Autodesk Inventor part; units mm, degrees
(part 3 of 3)
  line L522 (9.5, 12.75) -> (20, 12.75)
  line L523 (20, 12.75) -> (20, -5.25)
  line L524 (20, -5.25) -> (9.5, -5.25)
  line L525 (9.5, -5.25) -> (9.5, 12.75)
  line L526 (9.5, 17.25) -> (20, 17.25)
  line L527 (20, 17.25) -> (20, 35.25)
  line L528 (20, 35.25) -> (9.5, 35.25)
  line L529 (9.5, 35.25) -> (9.5, 17.25)
  line L530 (9.5, 57.75) -> (20, 57.75)
  line L531 (20, 57.75) -> (20, 39.75)
  line L532 (20, 39.75) -> (9.5, 39.75)
  line L533 (9.5, 39.75) -> (9.5, 57.75)
  line L534 (9.5, 62.25) -> (20, 62.25)
  line L535 (20, 62.25) -> (20, 80.25)
  line L536 (20, 80.25) -> (9.5, 80.25)
  line L537 (9.5, 80.25) -> (9.5, 62.25)
  line L538 (9.5, 117.75) -> (20, 117.75)
  line L539 (20, 117.75) -> (20, 99.75)
  line L540 (20, 99.75) -> (9.5, 99.75)
  line L541 (9.5, 99.75) -> (9.5, 117.75)
  line L542 (9.5, 84.75) -> (20, 84.75)
  line L543 (20, 84.75) -> (20, 95.25)
  line L544 (20, 95.25) -> (9.5, 95.25)
  line L545 (9.5, 95.25) -> (9.5, 84.75)
  point P0 (0, 0)
  point P1 (9.5, -64.25)
  point P2 (20, -53.75)
  point P3 (20, -49.25)
  point P4 (20, -8.75)
  point P5 (20, -4.25)
  point P6 (20, 36.25)
  point P7 (9.5, 40.75)
  point P8 (20, 51.25)
  point P9 (20, 55.75)
  point P10 (20, 96.25)
  point P11 (20, 100.75)
  point P12 (35, 27.75)
  point P13 (35, 17.25)
  point P14 (39.5, 17.25)
  point P15 (39.5, 27.75)
  point P16 (35, 42.75)
  point P17 (35, 57.75)
  point P18 (35, 72.75)
  point P19 (35, -47.25)
  point P20 (35, -77.25)
  point P21 (35, -32.25)
  point P22 (39.5, -32.25)
  point P23 (35, -17.25)
  point P24 (39.5, -17.25)
  point P25 (39.5, -12.75)
  point P26 (39.5, -2.25)
  point P27 (35, 12.75)
  point P28 (35, 2.25)
  point P29 (39.5, 2.25)
  point P30 (39.5, 12.75)
  point P31 (9.5, 99.75)
  point P32 (20, 99.75)
  point P33 (20, 102.75)
  point P34 (20, 107.25)
  point P35 (9.5, 107.25)
  point P36 (9.5, 102.75)
  point P37 (9.5, 95.25)
  point P38 (9.5, 92.25)
  point P39 (9.5, 87.75)
  point P40 (20, 84.75)
  point P41 (20, 87.75)
  point P42 (20, 92.25)
  point P43 (9.5, 80.25)
  point P44 (9.5, 77.25)
  point P45 (9.5, 72.75)
  point P46 (20, 72.75)
  point P47 (20, 77.25)
  point P48 (9.5, 39.75)
  point P49 (20, 42.75)
  point P50 (20, 47.25)
  point P51 (9.5, 47.25)
  point P52 (9.5, 42.75)
  point P53 (20, 35.25)
  point P54 (9.5, 35.25)
  point P55 (9.5, 32.25)
  point P56 (9.5, 27.75)
  point P57 (20, 27.75)
  point P58 (20, 32.25)
  point P59 (9.5, -5.25)
  point P60 (20, -5.25)
  point P61 (20, -2.25)
  point P62 (20, 2.25)
  point P63 (9.5, 2.25)
  point P64 (9.5, -2.25)
  point P65 (9.5, -9.75)
  point P66 (9.5, -12.75)
  point P67 (9.5, -17.25)
  point P68 (20, -20.25)
  point P69 (20, -17.25)
  point P70 (20, -12.75)
  point P71 (9.5, -24.75)
  point P72 (9.5, -27.75)
  point P73 (9.5, -32.25)
  point P74 (20, -32.25)
  point P75 (20, -27.75)
  point P76 (9.5, -65.25)
  point P77 (20, -62.25)
  point P78 (20, -57.75)
  point P79 (9.5, -57.75)
  point P80 (9.5, -62.25)
  point P81 (9.5, -69.75)
  point P82 (9.5, -72.75)
  point P83 (9.5, -77.25)
  point P84 (20, -77.25)
  point P85 (20, -72.75)
  dimension "d223" = 0.25
  dimension "d224" = 10.5
  dimension "d225" = 10.5
  dimension "d226" = 0.25
  dimension "d229" = 15
  dimension "d232" = 15
  dimension "d283" = 10.5
  dimension "d284" = 18
  dimension "d285" = 18
  dimension "d286" = 18
  dimension "d287" = 10.5
  dimension "d288" = 4.5
  dimension "d289" = 18
  dimension "d290" = 18
  dimension "d291" = 18
  dimension "d292" = 18
  dimension "d293" = 18
  dimension "d294" = 10.5
  dimension "d295" = 4.5
  constraints: 1088 end point, 50 parallel, 26 horizontal, 25 perpendicular, 21 point on line, 2 collinear, 1 vertical, 886 other
  measures "d223" distance between parallel lines of L4 L0
  measures "d224" distance of L0.start L0.end
  measures "d225" distance of L0.end L1.end
  measures "d226" distance between parallel lines of L5 L3
  measures "d229" distance of L0.start L6.start
  measures "d232" distance of L0.start L66.start
  measures "d283" distance of L508.end L507.end
  measures "d284" distance of L507.end L506.end
  measures "d285" distance of L510.end L511.end
  measures "d286" distance of L514.end L515.end
  measures "d287" distance of L518.end L519.end
  measures "d288" distance between parallel lines of L516 L518
  measures "d289" distance of L522.end L523.end
  measures "d290" distance of L526.end L527.end
  measures "d291" distance of L530.end L531.end
  measures "d292" distance of L534.end L535.end
  measures "d293" distance of L538.end L539.end
  measures "d294" distance of L542.end L543.end
  measures "d295" distance between parallel lines of L536 L542
extrude "Extrusion8" add sketch "Sketch21" along normal blind 1 contours L0 L1 L2 L3 | L6 L7 L8 L9 | L66 L67 L68 L69 | L70 L71 L72 L73 | L130 L131 L132 L133 | L134 L135 L136 L137 | L162 L163 L164 L165 | L166 L167 L168 L169 | L170 L171 L172 L173 | L174 L175 L176 L177 | L178 L179 L180 L181 | L182 L183 L184 L185 | L186 L187 L188 L189 | L190 L191 L192 L193 | L194 L195 L196 L197 | L198 L199 L200 L201 | L226 L227 L228 L229 | L230 L231 L232 L233 | L234 L235 L236 L237 | L238 L239 L240 L241 | L242 L243 L244 L245 | L246 L247 L248 L249 | L250 L251 L252 L253 | L254 L255 L256 L257 | L258 L259 L260 L261 | L262 L263 L264 L265 | L266 L267 L268 L269 | L268 L509 L270 L507 | L270 L271 L508 L273 | L512 L271 L272 L273 | L272 L513 L274 L511 | L274 L275 L276 L277 | L278 L279 L280 L281 | L280 L517 L282 L515 | L282 L283 L516 L285 | L518 L283 L284 L285 | L284 L521 L286 L519 | L286 L287 L520 L289 | L524 L287 L288 L289 | L288 L525 L290 L523 | L290 L291 L292 L293 | L294 L295 L296 L297 | L296 L529 L298 L527 | L298 L299 L528 L301 | L532 L299 L300 L301 | L300 L533 L302 L531 | L302 L303 L304 L305 | L306 L307 L308 L309 | L308 L537 L310 L535 | L310 L311 L536 L313 | L542 L311 L312 L313 | L312 L545 L314 L543 | L314 L315 L544 L317 | L540 L315 L316 L317 | L316 L541 L318 L539 | L318 L319 L320 L321 | L322 L323 L324 L325 | L326 L327 L328 L329 | L330 L331 L332 L333 | L333 L452 L395 L450 | L395 L396 L397 L394 | L334 L335 L336 L337 | L337 L456 L399 L454 | L399 L400 L401 L398 | L338 L339 L340 L341 | L341 L460 L403 L458 | L403 L404 L405 L402 | L342 L343 L344 L345 | L345 L464 L407 L462 | L407 L408 L409 L406 | L346 L347 L348 L349 | L349 L468 L411 L466 | L411 L412 L413 L410 | L350 L351 L352 L353 | L353 L472 L415 L470 | L415 L416 L417 L414 | L354 L355 L356 L357 | L357 L476 L419 L474 | L419 L420 L421 L418 | L358 L359 L360 L361 | L361 L480 L423 L478 | L423 L424 L425 L422 | L362 L363 L364 L365 | L365 L484 L427 L482 | L427 L428 L429 L426 | L366 L367 L368 L369 | L369 L488 L431 L486 | L431 L432 L433 L430 | L370 L371 L372 L373 | L373 L492 L435 L490 | L435 L436 L437 L434 | L374 L375 L376 L377 | L377 L496 L439 L494 | L439 L440 L441 L438 | L378 L379 L380 L381 | L381 L500 L443 L498 | L443 L444 L445 L442 | L382 L383 L384 L385 | L385 L504 L447 L502 | L447 L448 L449 L446 | L386 L387 L388 L389 | L390 L391 L392 L393
sketch "Sketch23" plane through (0, 4, 0) normal (0, 1, 0) x (1, 0, 0)
  circle A0 centre (-63.5, -131.25) radius 10.25
  line L0 (-60.5, 128.25) -> (-60.5, -128.25) projected
  line L1 (-60.5, -128.25) -> (60.5, -128.25) projected
  circle A1 centre (63.5, 131.25) radius 10.25
  circle A2 centre (63.5, -131.25) radius 10.25
  line L2 (60.5, -128.25) -> (60.5, 128.25) projected
  line L3 (60.5, 128.25) -> (-60.5, 128.25) projected
  circle A3 centre (-63.5, 131.25) radius 10.25
  circle A4 centre (-63.5, 0) radius 5.25
  circle A5 centre (63.5, 0) radius 5.25
  point P0 (0, 0)
  point P1 (-53.6989, -128.25)
  point P2 (-60.5, -121.4489)
  dimension "d338" = 20.5
  dimension "d339" = 3
  dimension "d340" = 3
  dimension "d341" = 20.5
  dimension "d342" = 3
  dimension "d343" = 3
  dimension "d344" = 20.5
  dimension "d345" = 3
  dimension "d346" = 3
  dimension "d347" = 3
  dimension "d348" = 3
  dimension "d349" = 20.5
  dimension "d350" = 10.5
  dimension "d351" = 3
  dimension "d352" = 128.25
  dimension "d353" = 10.5
  dimension "d354" = 3
  dimension "d355" = 128.25
  constraints: 6 centre point
  measures "d338" diameter of A0
  measures "d339" distance from line of L0 A0.centre
  measures "d340" distance from line of A0.centre L1
  measures "d341" diameter of A2
  measures "d342" distance from line of L2 A2.centre
  measures "d343" distance from line of L1 A2.centre
  measures "d344" diameter of A1
  measures "d345" distance from line of L3 A1.centre
  measures "d346" distance from line of L2 A1.centre
  measures "d347" distance from line of L0 A3.centre
  measures "d348" distance from line of L3 A3.centre
  measures "d349" diameter of A3
  measures "d350" diameter of A4
  measures "d351" distance from line of L0 A4.centre
  measures "d352" distance from line of L3 A4.centre
  measures "d353" diameter of A5
  measures "d354" distance from line of L2 A5.centre
  measures "d355" distance from line of L1 A5.centre
extrude "Extrusion9" cut sketch "Sketch23" against normal through all contours L1 L0 A0 | A2 L2 L1 | L1 L2 A2 | A4 L0 | L0 A4 | A5 L2 | L2 A5 | A3 L3 L0 | L0 L3 A3 | L2 L3 A1 | A1 L3 L2 picked at (-59.7398, -124.0546)
sketch "Sketch24" plane through (0, 4, 0) normal (0, 1, 0) x (1, 0, 0)
  line L0 (-52, 0.5) -> (-23, 0.5)
  line L1 (-23, 0.5) -> (-23, 29.5) construction
  line L2 (-23, 29.5) -> (-52, 29.5)
  line L3 (-52, 29.5) -> (-52, 0.5) construction
  line L4 (-52, 30.5) -> (-23, 30.5)
  line L5 (-23, 30.5) -> (-23, 59.5)
  line L6 (-23, 59.5) -> (-52, 59.5)
  line L7 (-52, 59.5) -> (-52, 30.5)
  line L8 (-52, 60.5) -> (-23, 60.5)
  line L9 (-23, 60.5) -> (-23, 89.5)
  line L10 (-23, 89.5) -> (-52, 89.5)
  line L11 (-52, 89.5) -> (-52, 60.5)
  line L12 (-52, 90.5) -> (-23, 90.5)
  line L13 (-23, 90.5) -> (-23, 119.5)
  line L14 (-23, 119.5) -> (-52, 119.5)
  line L15 (-52, 119.5) -> (-52, 90.5)
  line L16 (-60.5, 121.4489) -> (-60.5, 4.3084) projected
  line L17 (-43.5, 9) -> (-31.5, 9) construction
  line L18 (-31.5, 9) -> (-31.5, 21) construction
  line L19 (-31.5, 21) -> (-43.5, 21) construction
  line L20 (-43.5, 21) -> (-43.5, 9)
  line L21 (-43.5, 39) -> (-31.5, 39)
  line L22 (-31.5, 39) -> (-31.5, 51)
  line L23 (-31.5, 51) -> (-43.5, 51)
  line L24 (-43.5, 51) -> (-43.5, 39)
  line L25 (-43.5, 69) -> (-31.5, 69)
  line L26 (-31.5, 69) -> (-31.5, 81)
  line L27 (-31.5, 81) -> (-43.5, 81)
  line L28 (-43.5, 81) -> (-43.5, 69)
  line L29 (-43.5, 99) -> (-31.5, 99)
  line L30 (-31.5, 99) -> (-31.5, 111)
  line L31 (-31.5, 111) -> (-43.5, 111)
  line L32 (-43.5, 111) -> (-43.5, 99)
  line L33 (-49.7, 0.1) -> (-43.5, 0.1)
  line L34 (-43.5, 0.1) -> (-43.5, 26.3)
  line L35 (-43.5, 26.3) -> (-49.7, 26.3)
  line L36 (-49.7, 26.3) -> (-49.7, 0.1)
  line L37 (-49.7, 30.1) -> (-43.5, 30.1)
  line L38 (-43.5, 30.1) -> (-43.5, 56.3)
  line L39 (-43.5, 56.3) -> (-49.7, 56.3)
  line L40 (-49.7, 56.3) -> (-49.7, 30.1)
  line L41 (-49.7, 60.1) -> (-43.5, 60.1)
  line L42 (-43.5, 60.1) -> (-43.5, 86.3)
  line L43 (-43.5, 86.3) -> (-49.7, 86.3)
  line L44 (-49.7, 86.3) -> (-49.7, 60.1)
  line L45 (-49.7, 90.1) -> (-43.5, 90.1)
  line L46 (-43.5, 90.1) -> (-43.5, 116.3)
  line L47 (-43.5, 116.3) -> (-49.7, 116.3)
  line L48 (-49.7, 116.3) -> (-49.7, 90.1)
  line L49 (-31.5, 26.3) -> (-27.5, 26.3)
  line L50 (-27.5, 26.3) -> (-27.5, 6.3)
  line L51 (-27.5, 6.3) -> (-31.5, 6.3)
  line L52 (-31.5, 6.3) -> (-31.5, 26.3)
  line L53 (-31.5, 36.3) -> (-27.5, 36.3)
  line L54 (-27.5, 36.3) -> (-27.5, 56.3)
  line L55 (-27.5, 56.3) -> (-31.5, 56.3)
  line L56 (-31.5, 56.3) -> (-31.5, 36.3)
  line L57 (-31.5, 66.3) -> (-27.5, 66.3)
  line L58 (-27.5, 66.3) -> (-27.5, 86.3)
  line L59 (-27.5, 86.3) -> (-31.5, 86.3)
  line L60 (-31.5, 86.3) -> (-31.5, 66.3)
  line L61 (-31.5, 96.3) -> (-27.5, 96.3)
  line L62 (-27.5, 96.3) -> (-27.5, 116.3)
  line L63 (-27.5, 116.3) -> (-31.5, 116.3)
  line L64 (-31.5, 116.3) -> (-31.5, 96.3)
  line L65 (53.6989, 128.25) -> (-53.6989, 128.25) projected
  point P0 (0, 0)
  point P1 (-49.7, 90.5)
  point P2 (-43.5, 90.5)
  point P3 (-43.5, 111)
  point P4 (-49.7, 60.5)
  point P5 (-43.5, 60.5)
  point P6 (-43.5, 69)
  point P7 (-43.5, 81)
  point P8 (-49.7, 30.5)
  point P9 (-43.5, 30.5)
  point P10 (-43.5, 9)
  point P11 (-31.5, 39)
  point P12 (-31.5, 81)
  point P13 (-31.5, 111)
  dimension "d358" = 29
  dimension "d359" = 29
  dimension "d360" = 29
  dimension "d361" = 29
  dimension "d362" = 29
  dimension "d363" = 29
  dimension "d364" = 29
  dimension "d365" = 8.5
  dimension "d366" = 1
  dimension "d367" = 1
  dimension "d368" = 1
  dimension "d370" = 12
  dimension "d371" = 12
  dimension "d372" = 12
  dimension "d373" = 12
  dimension "d374" = 12
  dimension "d375" = 8.5
  dimension "d376" = 8.5
  dimension "d377" = 8.5
  dimension "d378" = 8.5
  dimension "d379" = 8.5
  dimension "d380" = 6.2
  dimension "d381" = 0
  dimension "d382" = 26.2
  dimension "d383" = 5.3
  dimension "d384" = 6.2
  dimension "d385" = 26.2
  dimension "d386" = 5.3
  dimension "d387" = 6.2
  dimension "d388" = 0
  dimension "d389" = 26.2
  dimension "d390" = 5.3
  dimension "d391" = 0
  dimension "d392" = 6.2
  dimension "d393" = 26.2
  dimension "d394" = 5.3
  dimension "d397" = 5.3
  dimension "d398" = 20
  dimension "d399" = 4
  dimension "d400" = 0
  dimension "d401" = 4
  dimension "d402" = 20
  dimension "d403" = 20
  dimension "d404" = 20
  dimension "d405" = 5.3
  dimension "d406" = 5.3
  dimension "d407" = 5.3
  dimension "d408" = 0
  dimension "d422" = 8.75
  constraints: 128 end point, 32 parallel, 16 horizontal, 16 perpendicular, 15 point on line
  measures "d358" distance of L0.end L1.end
  measures "d359" distance of L1.end L2.end
  measures "d360" distance of L5.end L6.end
  measures "d361" distance of L4.end L5.end
  measures "d362" distance of L8.end L9.end
  measures "d363" distance of L13.end L14.end
  measures "d364" distance of L12.end L13.end
  measures "d365" distance between parallel lines of L16 L3
  measures "d366" distance between parallel lines of L2 L4
  measures "d367" distance between parallel lines of L6 L8
  measures "d368" distance between parallel lines of L10 L12
  measures "d370" distance of L19.end L17.start
  measures "d371" distance of L18.end L19.end
  measures "d372" distance of L23.end L21.start
  measures "d373" distance of L27.end L25.start
  measures "d374" distance of L31.end L29.start
  measures "d375" distance between parallel lines of L3 L20
  measures "d376" distance between parallel lines of L2 L19
  measures "d377" distance between parallel lines of L4 L21
  measures "d378" distance between parallel lines of L8 L25
  measures "d379" distance between parallel lines of L12 L29
  measures "d380" distance of L34.end L35.end
  measures "d381" distance between parallel lines of L20 L34
  measures "d382" distance of L35.end L33.start
  measures "d383" distance between parallel lines of L19 L35
  measures "d384" distance of L46.end L47.end
  measures "d385" distance of L39.end L37.start
  measures "d386" distance between parallel lines of L39 L23
  measures "d387" distance of L38.end L39.end
  measures "d388" distance between parallel lines of L24 L38
  measures "d389" distance of L41.end L42.end
  measures "d390" distance between parallel lines of L27 L43
  measures "d391" distance between parallel lines of L28 L42
  measures "d392" distance of L42.end L43.end
  measures "d393" distance of L47.end L45.start
  measures "d394" distance between parallel lines of L31 L47
  measures "d397" distance between parallel lines of L19 L49
  measures "d398" distance of L49.end L50.end
  measures "d399" distance of L49.start L49.end
  measures "d400" distance between parallel lines of L18 L52
  measures "d401" distance of L54.end L55.end
  measures "d402" distance of L53.end L54.end
  measures "d403" distance of L57.end L58.end
  measures "d404" distance of L61.end L62.end
  measures "d405" distance between parallel lines of L31 L63
  measures "d406" distance between parallel lines of L27 L59
  measures "d407" distance between parallel lines of L23 L55
  measures "d408" distance between parallel lines of L22 L56
  measures "d422" distance between parallel lines of L65 L14
extrude "Extrusion10" add sketch "Sketch24" along normal blind 2.4 contours L36 L35 L34 L20 L0 | L0 L34 L33 L36 | L40 L39 L38 L24 L4 | L22 L56 L55 L54 L53 | L44 L43 L42 L28 L8 | L26 L60 L59 L58 L57 | L48 L47 L46 L32 L12 | L30 L64 L63 L62 L61 | L49 L50 L51 L52
sketch "Sketch25" plane through (0, 6.4, 0) normal (0, 1, 0) x (1, 0, 0)
  circle A0 centre (-46.15, 3.9) radius 1.5 projected
  circle A1 centre (-46.15, 20.6) radius 1.5 projected
  circle A2 centre (-46.15, 33.9) radius 1.5 projected
  circle A3 centre (-46.15, 50.6) radius 1.5 projected
  circle A4 centre (-46.15, 63.9) radius 1.5 projected
  circle A5 centre (-46.15, 80.6) radius 1.5 projected
  circle A6 centre (-46.15, 93.9) radius 1.5 projected
  circle A7 centre (-46.15, 110.6) radius 1.5 projected
  point P0 (0, 0)
  constraints: 8 coincident
hole "Hole1" at (-46.15, 6.4, -33.9) at (-46.15, 6.4, -50.6) at (-46.15, 6.4, -20.6) at (-46.15, 6.4, -3.9) at (-46.15, 6.4, -63.9) at (-46.15, 6.4, -80.6) at (-46.15, 6.4, -93.9) at (-46.15, 6.4, -110.6) direction (0, -1, 0) diameter 2.2 end through all
sketch "Sketch27" plane through (0, 4, 0) normal (0, 1, 0) x (1, 0, 0)
  line L0 (-43.5, 0.1) -> (-43.5, 26.3) projected
  line L1 (-27.5, 6.3) -> (-27.5, 26.3) projected
  line L2 (-43.5, 0.1) -> (-27.5, 0.1)
  line L3 (-27.5, 0.1) -> (-27.5, 6.3)
  line L4 (-27.5, 6.3) -> (-43.5, 6.3)
  line L5 (-43.5, 6.3) -> (-43.5, 0.1)
  line L6 (-43.5, 30.5) -> (-43.5, 56.3) projected
  line L7 (-27.5, 36.3) -> (-27.5, 56.3) projected
  line L8 (-43.5, 30.5) -> (-27.5, 30.5)
  line L9 (-27.5, 30.5) -> (-27.5, 36.3)
  line L10 (-27.5, 36.3) -> (-43.5, 36.3)
  line L11 (-43.5, 36.3) -> (-43.5, 30.5)
  line L12 (-43.5, 60.5) -> (-43.5, 86.3) projected
  line L13 (-31.5, 66.3) -> (-27.5, 66.3) projected
  line L14 (-43.5, 60.5) -> (-27.5, 60.5)
  line L15 (-27.5, 60.5) -> (-27.5, 66.3)
  line L16 (-27.5, 66.3) -> (-43.5, 66.3)
  line L17 (-43.5, 66.3) -> (-43.5, 60.5)
  line L18 (-43.5, 90.5) -> (-43.5, 116.3) projected
  line L19 (-31.5, 96.3) -> (-27.5, 96.3) projected
  line L20 (-43.5, 90.5) -> (-27.5, 90.5)
  line L21 (-27.5, 90.5) -> (-27.5, 96.3)
  line L22 (-27.5, 96.3) -> (-43.5, 96.3)
  line L23 (-43.5, 96.3) -> (-43.5, 90.5)
  line L24 (-60.5, 121.4489) -> (-60.5, 4.3084) projected
  line L25 (53.6989, 128.25) -> (-53.6989, 128.25) projected
  line L26 (-60.5, 120.75) -> (-19.75, 120.75)
  line L27 (-19.75, 120.75) -> (-19.75, 128.25)
  line L28 (-19.75, 128.25) -> (-60.5, 128.25)
  line L29 (-60.5, 128.25) -> (-60.5, 120.75)
  line L30 (-52.75, 123.75) -> (-22.75, 123.75) projected
  line L31 (-22.75, 123.75) -> (-22.75, 131.25) projected
  line L32 (-52.75, 131.25) -> (-22.75, 131.25) projected
  line L33 (-52.75, 123.75) -> (-52.75, 131.25) projected
  line L34 (-52.75, -131.25) -> (-22.75, -131.25) projected
  line L35 (-22.75, -131.25) -> (-22.75, -123.75) projected
  line L36 (-52.75, -123.75) -> (-22.75, -123.75) projected
  line L37 (-52.75, -131.25) -> (-52.75, -123.75) projected
  line L38 (-60.5, -4.3084) -> (-60.5, -121.4489) projected
  line L39 (-53.6989, -128.25) -> (53.6989, -128.25) projected
  line L40 (-60.5, -120.75) -> (-19.75, -120.75)
  line L41 (-19.75, -120.75) -> (-19.75, -128.25)
  line L42 (-19.75, -128.25) -> (-60.5, -128.25)
  line L43 (-60.5, -128.25) -> (-60.5, -120.75)
  point P0 (0, 0)
  point P1 (-53.6989, 128.25)
  dimension "d435" = 3
  dimension "d436" = 3
  dimension "d437" = 3
  dimension "d438" = 3
  constraints: 48 end point, 12 parallel, 6 horizontal, 6 perpendicular, 4 point on line
  measures "d435" distance between parallel lines of L27 L31
  measures "d436" distance between parallel lines of L30 L26
  measures "d437" distance between parallel lines of L40 L36
  measures "d438" distance between parallel lines of L41 L35
extrude "Extrusion11" cut sketch "Sketch27" against normal through all contours L0 L4 L3 L2 | L6 L10 L9 L8 | L12 L16 L13 L15 L14 | L18 L22 L19 L21 L20 | L29 L28 L25 L33 L30 L31 L27 L26 L24 | L25 L31 L30 L33 | L39 L42 L43 L38 L40 L41 L35 L36 L37 | L37 L36 L35 L39
sketch "Sketch28" plane through (0, 4, 0) normal (0, 1, 0) x (1, 0, 0)
  line L0 (-50.75, -88) -> (-50.75, -2) construction
  line L1 (5.25, -88) -> (-50.75, -88) construction
  line L2 (5.25, -2) -> (5.25, -88) construction
  line L3 (-50.75, -2) -> (5.25, -2) construction
  line L4 (-52.25, -1.5) -> (-52.25, -88.5)
  line L5 (-51.25, -89.5) -> (5.75, -89.5)
  line L6 (6.75, -88.5) -> (6.75, -1.5)
  line L7 (5.75, -0.5) -> (-51.25, -0.5)
  line L8 (-11, 0.5) -> (-19.5, 0.5) projected
  arc A0 (5.75, -89.5) -> (6.75, -88.5) centre (5.75, -88.5) ccw
  arc A1 (6.75, -1.5) -> (5.75, -0.5) centre (5.75, -1.5) ccw
  arc A2 (-51.25, -0.5) -> (-52.25, -1.5) centre (-51.25, -1.5) ccw
  arc A3 (-52.25, -88.5) -> (-51.25, -89.5) centre (-51.25, -88.5) ccw
  line L9 (5.25, -88) -> (-50.75, -88) projected
  point P0 (0, 0)
  dimension "d430" = 1
  dimension "d431" = 1
  constraints: 8 end point, 8 point on circle, 8 tangent, 4 centre point, 3 equal radius, 3 other
  measures "d430" distance between parallel lines of L7 L8
  measures "d431" radius of A0
extrude "Extrusion12" add sketch "Sketch28" along normal blind 20.3
sketch "Sketch30" plane through (0, 0, 0) normal (0, -1, 0) x (1, 0, 0)
  line L0 (-50.75, 2) -> (5.25, 2) construction
  line L1 (5.25, 2) -> (5.25, 88) construction
  line L2 (5.25, 88) -> (-50.75, 88) construction
  line L3 (-50.75, 88) -> (-50.75, 2) construction
  arc A0 (-51.25, 89.5) -> (-52.25, 88.5) centre (-51.25, 88.5) ccw projected
  line L4 (-51.25, 89.5) -> (5.75, 89.5) projected
  arc A1 (6.75, 88.5) -> (5.75, 89.5) centre (5.75, 88.5) ccw projected
  line L5 (6.75, 88.5) -> (6.75, 1.5) projected
  arc A2 (5.75, 0.5) -> (6.75, 1.5) centre (5.75, 1.5) ccw projected
  line L6 (5.75, 0.5) -> (-51.25, 0.5) projected
  arc A3 (-52.25, 1.5) -> (-51.25, 0.5) centre (-51.25, 1.5) ccw projected
  line L7 (-52.25, 1.5) -> (-52.25, 88.5) projected
  line L8 (-51, 1.75) -> (5.5, 1.75)
  line L9 (5.5, 1.75) -> (5.5, 88.25)
  line L10 (5.5, 88.25) -> (-51, 88.25)
  line L11 (-51, 88.25) -> (-51, 1.75)
  point P0 (0, 0)
  dimension "d439" = 1.5
  dimension "d440" = 1.5
  dimension "d441" = 1.5
  dimension "d442" = 1.5
  dimension "d443" = 0.25
  constraints: 16 end point, 4 parallel, 2 perpendicular, 1 horizontal, 3 other
  measures "d439" distance between parallel lines of L5 L1
  measures "d440" distance between parallel lines of L6 L0
  measures "d441" distance between parallel lines of L7 L3
  measures "d442" distance between parallel lines of L4 L2
  measures "d443" distance between parallel lines of L3 L11
extrude "Extrusion13" cut sketch "Sketch30" against normal through all contours L11 L10 L9 L8
sketch "Sketch31" plane through (0, 0, 0) normal (0, -1, 0) x (1, 0, 0)
  line L0 (5.25, 63) -> (-50.75, 63) projected
  line L1 (-51, 1.75) -> (-51, 88.25) projected
  line L2 (5.5, 88.25) -> (-51, 88.25) projected
  line L3 (-51, 63) -> (5.5, 63)
  line L4 (5.5, 63) -> (5.5, 88.25)
  line L5 (5.5, 88.25) -> (-51, 88.25)
  line L6 (-51, 88.25) -> (-51, 63)
  line L7 (5.5, 88.25) -> (5.5, 1.75) projected
  line L8 (5.5, 1.75) -> (-34.5, 1.75)
  line L9 (-34.5, 1.75) -> (-34.5, 5.75)
  line L10 (-34.5, 5.75) -> (5.5, 5.75)
  line L11 (5.5, 5.75) -> (5.5, 1.75)
  point P0 (0, 0)
  dimension "d446" = 4
  dimension "d447" = 40
  constraints: 16 end point, 4 parallel, 2 horizontal, 2 perpendicular, 2 point on line
  measures "d446" distance of L8.end L9.end
  measures "d447" distance between parallel lines of L7 L9
ref_plane "Work Plane1" through (-53.15, 15.8, 63) normal (0, -1, 0) x (1, 0, 0)
extrude "Extrusion14" add sketch "Sketch31" against normal up to surface (15.8 mm away)
sketch "Sketch32" plane through (0, 24.3, 0) normal (0, 1, 0) x (1, 0, 0)
  line L0 (-51.25, -89.5) -> (5.75, -89.5) projected
  arc A0 (5.75, -89.5) -> (6.75, -88.5) centre (5.75, -88.5) ccw projected
  line L1 (6.75, -88.5) -> (6.75, -1.5) projected
  arc A1 (6.75, -1.5) -> (5.75, -0.5) centre (5.75, -1.5) ccw projected
  line L2 (5.75, -0.5) -> (-51.25, -0.5) projected
  arc A2 (-51.25, -0.5) -> (-52.25, -1.5) centre (-51.25, -1.5) ccw projected
  line L3 (-52.25, -1.5) -> (-52.25, -88.5) projected
  arc A3 (-52.25, -88.5) -> (-51.25, -89.5) centre (-51.25, -88.5) ccw projected
  line L4 (5.25, -2) -> (5.25, -88) projected
  line L5 (-50.75, -2) -> (5.25, -2) projected
  line L6 (-50.75, -88) -> (-50.75, -2) projected
  line L7 (5.25, -88) -> (-50.75, -88) projected
  line L8 (-46.75, -5) -> (1.25, -5)
  line L9 (2.25, -6) -> (2.25, -84)
  line L10 (1.25, -85) -> (-46.75, -85)
  line L11 (-47.75, -84) -> (-47.75, -6)
  arc A4 (-47.75, -84) -> (-46.75, -85) centre (-46.75, -84) ccw
  arc A5 (-46.75, -5) -> (-47.75, -6) centre (-46.75, -6) ccw
  arc A6 (2.25, -6) -> (1.25, -5) centre (1.25, -6) ccw
  arc A7 (1.25, -85) -> (2.25, -84) centre (1.25, -84) ccw
  point P0 (0, 0)
  dimension "d450" = 3
  dimension "d451" = 1
  constraints: 8 end point, 8 point on circle, 8 tangent, 4 centre point, 3 equal radius, 3 other
  measures "d450" distance between parallel lines of L6 L11
  measures "d451" radius of A4
extrude "Extrusion15" add sketch "Sketch32" against normal blind 0.75 contours A3 L3 A2 L2 A1 L1 A0 L0 | L4 L7 L6 L5
body "Solid1"
